Battery_3000mAh_Anastasi_11-11-2020 v2 (Autodesk Fusion 360 design; units mm, degrees)
Autodesk Fusion 360 part; units mm, degrees
sketch "Sketch1" plane through (0, 0, 0) normal (0, 0, 1) x (1, 0, 0)
  line L0 (0, 0) -> (99, 0)
  line L1 (99, 0) -> (99, 48.5)
  line L2 (99, 48.5) -> (0, 48.5)
  line L3 (0, 48.5) -> (0, 0)
  dimension "d1" = 99
  dimension "d2" = 48.5
  constraint horizontal L0
  constraint vertical L1
  constraint horizontal L2
  constraint vertical L3
  constraint coincident L0.start L3.end
  measures "d1" distance of L0.start L0.end
  measures "d2" distance of L0.start L2.end
extrude "Extrude1" add sketch "Sketch1" along normal blind 5.5 makes body 1
fillet "Fillet1" radius 2 4 edges at (49.5, 0, 5.5) (49.5, 0, 0) (49.5, 48.5, 5.5) (49.5, 48.5, 0) on bodies 1
sketch "Sketch2" plane through (0, 0, 5.5) normal (0, 0, 1) x (-1, 0, 0)
  line L0 (-99, -46.5) -> (0, -46.5)
  line L1 (0, -46.5) -> (0, -2)
  line L2 (0, -2) -> (-99, -2)
  line L3 (-99, -2) -> (-99, -46.5)
  line L4 (-99, -5) -> (-6, -5)
  line L5 (-6, -5) -> (-6, -43.5)
  line L6 (-6, -43.5) -> (-99, -43.5)
  line L7 (-99, -43.5) -> (-99, -5)
  line L8 (-99, -48.5) -> (0, -48.5)
  line L9 (0, 0) -> (-99, 0)
  dimension "d7" = 6
  dimension "d8" = 5
  dimension "d9" = 5
  constraint horizontal L4
  constraint vertical L5
  constraint horizontal L6
  constraint vertical L7
  constraint coincident L3 L4.start
  measures "d7" distance of L1 L5
  measures "d8" distance of L6 L8
  measures "d9" distance of L4 L9
surface "Extrude2" add extruded along (0, 0, 1) between 0 and -6 path "Sketch2" along L4 L5 L6 L7 separate body makes body 2
split "Split1" by bodies 2 bodies 1 makes body 3 at (2, 17.8333, 0)
